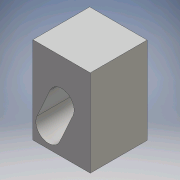
# Autodesk Inventor part: Part2
Saved by Autodesk Inventor 2016 (Build 200138000, 138)
## iProperties
Created: 2015-11-15
Part Number: Part2
Material: Generic
Document SubType Name: Modeling
Designer: Solomon
Density: 1 g/cm^3
Appearance: Default
Author: Solomon
Autodesk Inventor part; units mm, degrees
ref_plane "YZ Plane" through (0, 0, 0) normal (1, 0, 0) x (0, 1, 0)
ref_plane "XZ Plane" through (0, 0, 0) normal (0, 1, 0) x (-1, 0, 0)
ref_plane "XY Plane" through (0, 0, 0) normal (0, 0, 1) x (1, 0, 0)
sketch "Sketch1" plane through (0, 0, 0) normal (0, 1, 0) x (-1, 0, 0)
  line L0 (8.7498, 17.9442) -> (-1.3539, 17.9442)
  line L1 (-1.3539, 17.9442) -> (-1.3539, 2.6674)
  line L2 (-1.3539, 2.6674) -> (8.7498, 2.6674)
  line L3 (8.7498, 2.6674) -> (8.7498, 17.9442)
  line L4 (6.0139, 5.7417) -> (3.698, 10.8481) construction
  line L5 (8.0291, 6.6557) -> (5.7132, 11.7621)
  line L6 (1.6827, 9.9341) -> (3.9986, 4.8277)
  arc A0 (3.9986, 4.8277) -> (8.0291, 6.6557) centre (6.0139, 5.7417) ccw
  arc A1 (5.7132, 11.7621) -> (1.6827, 9.9341) centre (3.698, 10.8481) ccw
  point P0 (0, 0)
  point P1 (4.8559, 8.2949)
  constraints: 16 end point, 4 point on circle, 4 tangent, 3 parallel, 2 centre point, 1 horizontal, 1 midpoint, 1 perpendicular
extrude "Extrusion1" add sketch "Sketch1" along normal blind 10
body "Solid1"
